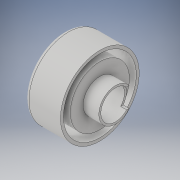
# Autodesk Inventor part: RearWheelLeft
Saved by Autodesk Inventor 2017 (Build 210142000, 142)
## iProperties
Created: 2017-08-21
Part Number: RearWheelLeft
Material: Generic
Document SubType Name: Modeling
Designer: MineV
Density: 1 g/cm^3
Appearance: Default
Author: MineV
Autodesk Inventor part; units mm, degrees
ref_plane "XZ Plane" through (0, 0, 0) normal (0, 1, 0) x (-1, 0, 0)
ref_plane "XY Plane" through (0, 0, 0) normal (0, 0, 1) x (1, 0, 0)
ref_plane "Work Plane1" through (20, 0, 0) normal (1, 0, 0) x (0, 1, 0)
sketch "Sketch7" plane through (0, 0, 0) normal (1, 0, 0) x (0, 1, 0)
  circle A0 centre (0, 0) radius 7.5
  circle A1 centre (0, 0) radius 20
  dimension "d28" = 15
  dimension "d29" = 40
  constraints: 2 centre point, 2 coincident
  measures "d28" diameter of A0
  measures "d29" diameter of A1
extrude "Wheel" add sketch "Sketch7" along normal blind 18
sketch "Sketch8" plane through (0, 0, 0) normal (1, 0, 0) x (0, 1, 0)
  circle A0 centre (0, 0) radius 8.5
  circle A1 centre (0, 0) radius 13.5
  dimension "d32" = 17
  dimension "d33" = 27
  constraints: 2 centre point, 2 coincident
  measures "d32" diameter of A0
  measures "d33" diameter of A1
extrude "Extrusion7" cut sketch "Sketch8" along normal blind 17
sketch "Sketch9" plane through (0, 0, 0) normal (-1, 0, 0) x (0, 0, 1)
  circle A0 centre (0, 0) radius 11.0642
  constraints: 1 centre point, 1 coincident
extrude "Extrusion8" cut sketch "Sketch9" against normal blind 3
fillet "Fillet1" radius 2 1 edges at (0, -20, 0)
fillet "Fillet2" radius 1 1 edges at (0, -13.5, 0)
shell "Shell1" thickness 1.5 removed faces 1 at (18, 15.6396, -1.5954)
sketch "Sketch10" plane through (18, 0, 0) normal (1, 0, 0) x (0, 0, -1)
  circle A0 centre (0, 0) radius 8.5
  circle A1 centre (0, 0) radius 7.5 projected
  dimension "d41" = 17
  constraints: 1 centre point, 1 coincident
  measures "d41" diameter of A0
extrude "Extrusion9" add sketch "Sketch10" along normal blind 8
sketch "Sketch11" plane through (0, 0, 0) normal (0, 0, 1) x (1, 0, 0)
  line L0 (26, -8.5) -> (26, 8.5) projected
  line L1 (18, 8.5) -> (18, -8.5) projected
  line L2 (26, 7.5) -> (26, -7.5) projected
  line L3 (26, -5) -> (23, -5)
  line L4 (23, -5) -> (23, 5)
  line L5 (23, 5) -> (26, 5)
  line L6 (26, 5) -> (26, -5)
  line L7 (0, 0) -> (9.4673, 0) construction
  dimension "d44" = 3
  dimension "d45" = 10
  dimension "d46" = 5
  constraints: 10 end point, 2 horizontal, 2 parallel, 1 perpendicular, 1 point on line
  measures "d44" distance of L4.end L5.end
  measures "d45" distance of L3.end L4.end
  measures "d46" distance between parallel lines of L7 L3
extrude "Extrusion10" cut sketch "Sketch11" against normal blind 20
equation "\"d46\" = 0.5 * d45"
body "Solid1"
